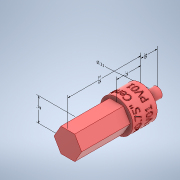
# Autodesk Inventor part: 1x8mmx1_75-inchHexShaft
Saved by Autodesk Inventor 2022.2 (Build 262287000, 287)
## iProperties
Created: 2020-11-16
Part Number: 1x8mmx1_75-inchHexShaft
Material: PC/ABS Plastic
Document SubType Name: Modeling
Designer: robst
Density: 0.357273 g/cm^3
Appearance: Smooth - Red
Author: robst
Autodesk Inventor part; units mm, degrees
ref_plane "XZ Plane" through (0, 0, 0) normal (0, 1, 0) x (-1, 0, 0)
ref_plane "XY Plane" through (0, 0, 0) normal (0, 0, 1) x (1, 0, 0)
sketch "Sketch1" plane through (0, 0, 0) normal (0, 0, 1) x (1, 0, 0)
  line L0 (10.9985, 0) -> (5.4993, -9.525)
  line L1 (5.4993, -9.525) -> (-5.4993, -9.525)
  line L2 (-5.4993, -9.525) -> (-10.9985, 0)
  line L3 (-10.9985, 0) -> (-5.4993, 9.525)
  line L4 (-5.4993, 9.525) -> (5.4993, 9.525)
  line L5 (5.4993, 9.525) -> (10.9985, 0)
  point P0 (0, 0)
  point P1 (0, 0)
  dimension "d0" = 19.05
  constraints: 12 end point, 1 coincident, 1 horizontal, 13 other
  measures "d0" distance between parallel lines of L1 L4
extrude "Hex Portion" add sketch "Sketch1" along normal mid plane 38.1
sketch "Sketch2" plane through (0, 0, -19.05) normal (0, 0, -1) x (-1, 0, 0)
  circle A0 centre (0, 0) radius 12.7
  dimension "d3" = 25.4
  constraints: 1 centre point, 1 coincident
  measures "d3" diameter of A0
extrude "Extrusion2" add sketch "Sketch2" along normal blind 19.05
thicken "Reduce Size of Hex Shaft" operation add thickness 0.1905 both sides no extend neighbours yes toward (-0.8660254, -0.5, 0) faces at (9.1654, 3.175, -6.35) (-1.8331, 9.525, 6.35) (7.3323, -6.35, -6.35) (-1.8331, -9.525, -6.35) (-7.3323, -6.35, 6.35) (-9.1654, 3.175, 6.35)
sketch "Sketch3" plane through (0, 0, -38.1) normal (0, 0, -1) x (-1, 0, 0)
  circle A0 centre (0, 0) radius 4
  dimension "d14" = 8
  constraints: 1 centre point, 1 coincident
  measures "d14" diameter of A0
extrude "Extrusion3" add sketch "Sketch3" along normal blind 12.7
ref_plane "Work Plane1" through (12.7, 0, -19.05) normal (1, 0, 0) x (0, 1, 0)
sketch "Sketch4" plane through (12.7, 0, -19.05) normal (1, 0, 0) x (0, 1, 0)
  line L0 (-12.7, 0) -> (12.7, 0) projected
  line L1 (-12.7, -19.05) -> (12.7, -19.05) projected
  line L2 (-12.7, 0) -> (-12.7, -19.05) construction
  line L3 (-12.7, -9.525) -> (12.7, -9.525) construction
  line L4 (12.7, 0) -> (12.7, -19.05) construction
  line L5 (-30.7085, -6.985) -> (-33.1867, -6.985)
  line L6 (-33.1867, -6.985) -> (-33.1867, -6.4663)
  line L7 (-33.1867, -6.4663) -> (-32.2646, -6.4663)
  line L8 (-32.2646, -6.4663) -> (-32.2646, -3.0618)
  line L9 (-32.2646, -3.0618) -> (-33.1867, -3.0618)
  line L10 (-33.1867, -3.0618) -> (-33.1867, -2.5966)
  spline S0 degree 2 poles (-33.1867, -2.5966) (-32.6639, -2.5966) (-32.1699, -2.3002) (-32.137, -1.8885) knots 0 0 0 1 2 2 2
  line L11 (-32.137, -1.8885) -> (-31.61, -1.8885)
  line L12 (-31.61, -1.8885) -> (-31.61, -6.4663)
  line L13 (-31.61, -6.4663) -> (-30.7085, -6.4663)
  line L14 (-30.7085, -6.4663) -> (-30.7085, -6.985)
  line L15 (-29.0124, -1.6786) -> (-29.1606, -3.6546)
  line L16 (-29.1606, -3.6546) -> (-29.6093, -3.6546)
  line L17 (-29.6093, -3.6546) -> (-29.7575, -1.6786)
  line L18 (-29.7575, -1.6786) -> (-29.0124, -1.6786)
  line L19 (-27.728, -1.6786) -> (-27.8762, -3.6546)
  line L20 (-27.8762, -3.6546) -> (-28.3249, -3.6546)
  line L21 (-28.3249, -3.6546) -> (-28.4731, -1.6786)
  line L22 (-28.4731, -1.6786) -> (-27.728, -1.6786)
  line L23 (-23.9159, -6.985) -> (-24.7022, -6.985)
  line L24 (-24.7022, -6.985) -> (-25.6285, -5.5524)
  line L25 (-25.6285, -5.5524) -> (-26.5794, -6.985)
  line L26 (-26.5794, -6.985) -> (-27.3081, -6.985)
  line L27 (-27.3081, -6.985) -> (-25.9866, -5.0954)
  line L28 (-25.9866, -5.0954) -> (-27.2957, -3.1729)
  line L29 (-27.2957, -3.1729) -> (-26.5095, -3.1729)
  line L30 (-26.5095, -3.1729) -> (-25.5873, -4.5932)
  line L31 (-25.5873, -4.5932) -> (-24.6446, -3.1729)
  line L32 (-24.6446, -3.1729) -> (-23.9159, -3.1729)
  line L33 (-23.9159, -3.1729) -> (-25.2292, -5.0543)
  line L34 (-25.2292, -5.0543) -> (-23.9159, -6.985)
  spline S1 degree 2 poles (-21.977, -7.1003) (-22.3557, -7.1003) (-22.9773, -6.8738) (-23.1955, -6.6639) knots 0 0 0 1 2 2 2
  spline S2 degree 2 poles (-23.1955, -6.6639) (-23.4096, -6.4581) (-23.6319, -5.8982) (-23.6319, -5.5812) knots 0 0 0 1 2 2 2
  spline S3 degree 2 poles (-23.6319, -5.5812) (-23.6319, -5.1695) (-23.1914, -4.4779) (-22.7715, -4.2721) knots 0 0 0 1 2 2 2
  line L35 (-22.7715, -4.2721) -> (-22.7715, -4.2515)
  spline S4 degree 2 poles (-22.7715, -4.2515) (-23.1461, -4.0333) (-23.5084, -3.5146) (-23.5084, -3.1277) knots 0 0 0 1 2 2 2
  spline S5 degree 2 poles (-23.5084, -3.1277) (-23.5084, -2.5554) (-22.6439, -1.7897) (-21.977, -1.7897) knots 0 0 0 1 2 2 2
  spline S6 degree 2 poles (-21.977, -1.7897) (-21.2854, -1.7897) (-20.4497, -2.5143) (-20.4497, -3.0824) knots 0 0 0 1 2 2 2
  spline S7 degree 2 poles (-20.4497, -3.0824) (-20.4497, -3.4241) (-20.849, -4.091) (-21.2236, -4.2803) knots 0 0 0 1 2 2 2
  line L36 (-21.2236, -4.2803) -> (-21.2236, -4.3009)
  spline S8 degree 2 poles (-21.2236, -4.3009) (-20.779, -4.5068) (-20.3221, -5.0996) (-20.3221, -5.5689) knots 0 0 0 1 2 2 2
  spline S9 degree 2 poles (-20.3221, -5.5689) (-20.3221, -6.2193) (-21.2689, -7.1003) (-21.977, -7.1003) knots 0 0 0 1 2 2 2
  spline S10 degree 2 poles (-21.0219, -5.6347) (-21.0219, -5.3219) (-21.2689, -4.9514) (-21.6188, -4.762) knots 0 0 0 1 2 2 2
  spline S11 degree 2 poles (-21.6188, -4.762) (-21.7341, -4.6961) (-22.1211, -4.5438) (-22.3639, -4.445) knots 0 0 0 1 2 2 2
  spline S12 degree 2 poles (-22.3639, -4.445) (-22.6439, -4.6303) (-22.9444, -5.1819) (-22.9444, -5.5318) knots 0 0 0 1 2 2 2
  spline S13 degree 2 poles (-22.9444, -5.5318) (-22.9444, -5.9929) (-22.3886, -6.5939) (-21.9687, -6.5939) knots 0 0 0 1 2 2 2
  spline S14 degree 2 poles (-21.9687, -6.5939) (-21.5406, -6.5939) (-21.0219, -6.0793) (-21.0219, -5.6347) knots 0 0 0 1 2 2 2
  spline S15 degree 2 poles (-21.1166, -3.0906) (-21.1166, -2.7489) (-21.5735, -2.292) (-21.9811, -2.292) knots 0 0 0 1 2 2 2
  spline S16 degree 2 poles (-21.9811, -2.292) (-22.3516, -2.292) (-22.825, -2.6995) (-22.825, -3.0494) knots 0 0 0 1 2 2 2
  spline S17 degree 2 poles (-22.825, -3.0494) (-22.825, -3.3006) (-22.5821, -3.6505) (-22.3392, -3.7904) knots 0 0 0 1 2 2 2
  spline S18 degree 2 poles (-22.3392, -3.7904) (-22.2363, -3.8481) (-21.8, -4.0498) (-21.6229, -4.1074) knots 0 0 0 1 2 2 2
  spline S19 degree 2 poles (-21.6229, -4.1074) (-21.3265, -3.881) (-21.1166, -3.3994) (-21.1166, -3.0906) knots 0 0 0 1 2 2 2
  line L37 (-15.2832, -6.985) -> (-15.2832, -4.7785)
  spline S20 degree 2 poles (-15.2832, -4.7785) (-15.2832, -4.515) (-15.3244, -4.0663) (-15.3903, -3.9428) knots 0 0 0 1 2 2 2
  spline S21 degree 2 poles (-15.3903, -3.9428) (-15.4561, -3.8069) (-15.7072, -3.6752) (-15.9254, -3.6752) knots 0 0 0 1 2 2 2
  spline S22 degree 2 poles (-15.9254, -3.6752) (-16.123, -3.6752) (-16.5759, -3.9181) (-16.8146, -4.1486) knots 0 0 0 1 2 2 2
  spline S23 degree 2 poles (-16.8146, -4.1486) (-16.8105, -4.2062) (-16.8023, -4.3668) (-16.8023, -4.4738) knots 0 0 0 1 2 2 2
  line L38 (-16.8023, -4.4738) -> (-16.8023, -6.985)
  line L39 (-16.8023, -6.985) -> (-17.4445, -6.985)
  line L40 (-17.4445, -6.985) -> (-17.4445, -4.7785)
  spline S24 degree 2 poles (-17.4445, -4.7785) (-17.4445, -4.515) (-17.4857, -4.0663) (-17.5515, -3.9428) knots 0 0 0 1 2 2 2
  spline S25 degree 2 poles (-17.5515, -3.9428) (-17.6174, -3.8069) (-17.8685, -3.6752) (-18.0867, -3.6752) knots 0 0 0 1 2 2 2
  spline S26 degree 2 poles (-18.0867, -3.6752) (-18.2925, -3.6752) (-18.7495, -3.9345) (-18.9636, -4.1362) knots 0 0 0 1 2 2 2
  line L41 (-18.9636, -4.1362) -> (-18.9636, -6.985)
  line L42 (-18.9636, -6.985) -> (-19.6058, -6.985)
  line L43 (-19.6058, -6.985) -> (-19.6058, -3.1729)
  line L44 (-19.6058, -3.1729) -> (-18.9636, -3.1729)
  line L45 (-18.9636, -3.1729) -> (-18.9636, -3.5928)
  spline S27 degree 2 poles (-18.9636, -3.5928) (-18.7124, -3.3417) (-18.2184, -3.0659) (-17.922, -3.0659) knots 0 0 0 1 2 2 2
  spline S28 degree 2 poles (-17.922, -3.0659) (-17.5845, -3.0659) (-17.0616, -3.3747) (-16.9258, -3.7246) knots 0 0 0 1 2 2 2
  spline S29 degree 2 poles (-16.9258, -3.7246) (-16.6335, -3.3994) (-16.0819, -3.0659) (-15.7608, -3.0659) knots 0 0 0 1 2 2 2
  spline S30 degree 2 poles (-15.7608, -3.0659) (-15.5138, -3.0659) (-15.1103, -3.2182) (-14.9621, -3.3911) knots 0 0 0 1 2 2 2
  spline S31 degree 2 poles (-14.9621, -3.3911) (-14.8098, -3.564) (-14.641, -4.0827) (-14.641, -4.4738) knots 0 0 0 1 2 2 2
  line L46 (-14.641, -4.4738) -> (-14.641, -6.985)
  line L47 (-14.641, -6.985) -> (-15.2832, -6.985)
  line L48 (-9.4169, -6.985) -> (-9.4169, -4.7785)
  spline S32 degree 2 poles (-9.4169, -4.7785) (-9.4169, -4.515) (-9.4581, -4.0663) (-9.524, -3.9428) knots 0 0 0 1 2 2 2
  spline S33 degree 2 poles (-9.524, -3.9428) (-9.5898, -3.8069) (-9.841, -3.6752) (-10.0591, -3.6752) knots 0 0 0 1 2 2 2
  spline S34 degree 2 poles (-10.0591, -3.6752) (-10.2567, -3.6752) (-10.7096, -3.9181) (-10.9483, -4.1486) knots 0 0 0 1 2 2 2
  spline S35 degree 2 poles (-10.9483, -4.1486) (-10.9442, -4.2062) (-10.936, -4.3668) (-10.936, -4.4738) knots 0 0 0 1 2 2 2
  line L49 (-10.936, -4.4738) -> (-10.936, -6.985)
  line L50 (-10.936, -6.985) -> (-11.5782, -6.985)
  line L51 (-11.5782, -6.985) -> (-11.5782, -4.7785)
  spline S36 degree 2 poles (-11.5782, -4.7785) (-11.5782, -4.515) (-11.6194, -4.0663) (-11.6852, -3.9428) knots 0 0 0 1 2 2 2
  spline S37 degree 2 poles (-11.6852, -3.9428) (-11.7511, -3.8069) (-12.0022, -3.6752) (-12.2204, -3.6752) knots 0 0 0 1 2 2 2
  spline S38 degree 2 poles (-12.2204, -3.6752) (-12.4262, -3.6752) (-12.8832, -3.9345) (-13.0973, -4.1362) knots 0 0 0 1 2 2 2
  line L52 (-13.0973, -4.1362) -> (-13.0973, -6.985)
  line L53 (-13.0973, -6.985) -> (-13.7395, -6.985)
  line L54 (-13.7395, -6.985) -> (-13.7395, -3.1729)
  line L55 (-13.7395, -3.1729) -> (-13.0973, -3.1729)
  line L56 (-13.0973, -3.1729) -> (-13.0973, -3.5928)
  spline S39 degree 2 poles (-13.0973, -3.5928) (-12.8461, -3.3417) (-12.3521, -3.0659) (-12.0557, -3.0659) knots 0 0 0 1 2 2 2
  spline S40 degree 2 poles (-12.0557, -3.0659) (-11.7182, -3.0659) (-11.1953, -3.3747) (-11.0595, -3.7246) knots 0 0 0 1 2 2 2
  spline S41 degree 2 poles (-11.0595, -3.7246) (-10.7672, -3.3994) (-10.2156, -3.0659) (-9.8945, -3.0659) knots 0 0 0 1 2 2 2
  spline S42 degree 2 poles (-9.8945, -3.0659) (-9.6475, -3.0659) (-9.244, -3.2182) (-9.0958, -3.3911) knots 0 0 0 1 2 2 2
  spline S43 degree 2 poles (-9.0958, -3.3911) (-8.9435, -3.564) (-8.7747, -4.0827) (-8.7747, -4.4738) knots 0 0 0 1 2 2 2
  line L57 (-8.7747, -4.4738) -> (-8.7747, -6.985)
  line L58 (-8.7747, -6.985) -> (-9.4169, -6.985)
  line L59 (-4.9133, -6.985) -> (-5.6996, -6.985)
  line L60 (-5.6996, -6.985) -> (-6.6258, -5.5524)
  line L61 (-6.6258, -5.5524) -> (-7.5768, -6.985)
  line L62 (-7.5768, -6.985) -> (-8.3054, -6.985)
  line L63 (-8.3054, -6.985) -> (-6.984, -5.0954)
  line L64 (-6.984, -5.0954) -> (-8.2931, -3.1729)
  line L65 (-8.2931, -3.1729) -> (-7.5068, -3.1729)
  line L66 (-7.5068, -3.1729) -> (-6.5847, -4.5932)
  line L67 (-6.5847, -4.5932) -> (-5.6419, -3.1729)
  line L68 (-5.6419, -3.1729) -> (-4.9133, -3.1729)
  line L69 (-4.9133, -3.1729) -> (-6.2265, -5.0543)
  line L70 (-6.2265, -5.0543) -> (-4.9133, -6.985)
  spline S44 degree 2 poles (-1.3482, -4.445) (-1.3482, -5.8117) (-2.1427, -7.092) (-2.9702, -7.092) knots 0 0 0 1 2 2 2
  spline S45 degree 2 poles (-2.9702, -7.092) (-3.81, -7.092) (-4.5963, -5.787) (-4.5963, -4.4491) knots 0 0 0 1 2 2 2
  spline S46 degree 2 poles (-4.5963, -4.4491) (-4.5963, -3.0741) (-3.8018, -1.8021) (-2.9702, -1.8021) knots 0 0 0 1 2 2 2
  spline S47 degree 2 poles (-2.9702, -1.8021) (-2.1345, -1.8021) (-1.3482, -3.1194) (-1.3482, -4.445) knots 0 0 0 1 2 2 2
  spline S48 degree 2 poles (-2.221, -5.9929) (-2.1222, -5.7418) (-2.0398, -4.9678) (-2.0398, -4.445) knots 0 0 0 1 2 2 2
  spline S49 degree 2 poles (-2.0398, -4.445) (-2.0398, -3.9222) (-2.1222, -3.1524) (-2.2251, -2.893) knots 0 0 0 1 2 2 2
  spline S50 degree 2 poles (-2.2251, -2.893) (-2.328, -2.6337) (-2.6861, -2.3661) (-2.9702, -2.3661) knots 0 0 0 1 2 2 2
  spline S51 degree 2 poles (-2.9702, -2.3661) (-3.2542, -2.3661) (-3.6206, -2.6337) (-3.7277, -2.9012) knots 0 0 0 1 2 2 2
  spline S52 degree 2 poles (-3.7277, -2.9012) (-3.8306, -3.1606) (-3.9047, -3.951) (-3.9047, -4.4491) knots 0 0 0 1 2 2 2
  spline S53 degree 2 poles (-3.9047, -4.4491) (-3.9047, -4.9843) (-3.8388, -5.7006) (-3.7318, -5.9805) knots 0 0 0 1 2 2 2
  spline S54 degree 2 poles (-3.7318, -5.9805) (-3.633, -6.244) (-3.2666, -6.528) (-2.9702, -6.528) knots 0 0 0 1 2 2 2
  spline S55 degree 2 poles (-2.9702, -6.528) (-2.6903, -6.528) (-2.3239, -6.2605) (-2.221, -5.9929) knots 0 0 0 1 2 2 2
  line L71 (0.3931, -6.985) -> (-0.422, -6.985)
  line L72 (-0.422, -6.985) -> (-0.422, -6.0135)
  line L73 (-0.422, -6.0135) -> (0.3931, -6.0135)
  line L74 (0.3931, -6.0135) -> (0.3931, -6.985)
  line L75 (4.6086, -2.6666) -> (2.4103, -6.985)
  line L76 (2.4103, -6.985) -> (1.6858, -6.985)
  line L77 (1.6858, -6.985) -> (4.0076, -2.5019)
  line L78 (4.0076, -2.5019) -> (1.3853, -2.5019)
  line L79 (1.3853, -2.5019) -> (1.3853, -1.905)
  line L80 (1.3853, -1.905) -> (4.6086, -1.905)
  line L81 (4.6086, -1.905) -> (4.6086, -2.6666)
  spline S56 degree 2 poles (8.3095, -5.3713) (8.3095, -5.7376) (8.0749, -6.3634) (7.8608, -6.5939) knots 0 0 0 1 2 2 2
  spline S57 degree 2 poles (7.8608, -6.5939) (7.6468, -6.8244) (7.0087, -7.092) (6.6135, -7.092) knots 0 0 0 1 2 2 2
  spline S58 degree 2 poles (6.6135, -7.092) (6.2512, -7.092) (5.5431, -6.9315) (5.2838, -6.8039) knots 0 0 0 1 2 2 2
  line L82 (5.2838, -6.8039) -> (5.2838, -6.0834)
  line L83 (5.2838, -6.0834) -> (5.3332, -6.0834)
  spline S59 degree 2 poles (5.3332, -6.0834) (5.4114, -6.1411) (5.7037, -6.2893) (5.8807, -6.3551) knots 0 0 0 1 2 2 2
  spline S60 degree 2 poles (5.8807, -6.3551) (6.0824, -6.4251) (6.4159, -6.5033) (6.6258, -6.5033) knots 0 0 0 1 2 2 2
  spline S61 degree 2 poles (6.6258, -6.5033) (6.8317, -6.5033) (7.2186, -6.3551) (7.3586, -6.1946) knots 0 0 0 1 2 2 2
  spline S62 degree 2 poles (7.3586, -6.1946) (7.4862, -6.0423) (7.6179, -5.6388) (7.6179, -5.3671) knots 0 0 0 1 2 2 2
  spline S63 degree 2 poles (7.6179, -5.3671) (7.6179, -5.0954) (7.4697, -4.7496) (7.3298, -4.6344) knots 0 0 0 1 2 2 2
  spline S64 degree 2 poles (7.3298, -4.6344) (7.1857, -4.5068) (6.7576, -4.3997) (6.4982, -4.3997) knots 0 0 0 1 2 2 2
  spline S65 degree 2 poles (6.4982, -4.3997) (6.2183, -4.3997) (5.6625, -4.4862) (5.4937, -4.5232) knots 0 0 0 1 2 2 2
  line L84 (5.4937, -4.5232) -> (5.4937, -1.905)
  line L85 (5.4937, -1.905) -> (8.2807, -1.905)
  line L86 (8.2807, -1.905) -> (8.2807, -2.5019)
  line L87 (8.2807, -2.5019) -> (6.1483, -2.5019)
  line L88 (6.1483, -2.5019) -> (6.1483, -3.8563)
  spline S66 degree 2 poles (6.1483, -3.8563) (6.2718, -3.8398) (6.5105, -3.8275) (6.6094, -3.8275) knots 0 0 0 1 2 2 2
  spline S67 degree 2 poles (6.6094, -3.8275) (7.0004, -3.8275) (7.5397, -3.9551) (7.7867, -4.1445) knots 0 0 0 1 2 2 2
  spline S68 degree 2 poles (7.7867, -4.1445) (8.0378, -4.3338) (8.3095, -4.9102) (8.3095, -5.3713) knots 0 0 0 1 2 2 2
  line L89 (9.8039, -1.6786) -> (9.6557, -3.6546)
  line L90 (9.6557, -3.6546) -> (9.207, -3.6546)
  line L91 (9.207, -3.6546) -> (9.0588, -1.6786)
  line L92 (9.0588, -1.6786) -> (9.8039, -1.6786)
  line L93 (11.0883, -1.6786) -> (10.9401, -3.6546)
  line L94 (10.9401, -3.6546) -> (10.4914, -3.6546)
  line L95 (10.4914, -3.6546) -> (10.3432, -1.6786)
  line L96 (10.3432, -1.6786) -> (11.0883, -1.6786)
  spline S69 degree 2 poles (16.156, -7.0756) (15.662, -7.0756) (14.8263, -6.7421) (14.5216, -6.4087) knots 0 0 0 1 2 2 2
  spline S70 degree 2 poles (14.5216, -6.4087) (14.217, -6.0793) (13.8835, -5.0913) (13.8835, -4.4491) knots 0 0 0 1 2 2 2
  spline S71 degree 2 poles (13.8835, -4.4491) (13.8835, -3.811) (14.2088, -2.8642) (14.5175, -2.5143) knots 0 0 0 1 2 2 2
  spline S72 degree 2 poles (14.5175, -2.5143) (14.8222, -2.1726) (15.6537, -1.8144) (16.1683, -1.8144) knots 0 0 0 1 2 2 2
  spline S73 degree 2 poles (16.1683, -1.8144) (16.4235, -1.8144) (16.8723, -1.8885) (17.0616, -1.9462) knots 0 0 0 1 2 2 2
  spline S74 degree 2 poles (17.0616, -1.9462) (17.2263, -1.9997) (17.568, -2.152) (17.7368, -2.2426) knots 0 0 0 1 2 2 2
  line L97 (17.7368, -2.2426) -> (17.7368, -3.0577)
  line L98 (17.7368, -3.0577) -> (17.6833, -3.0577)
  spline S75 degree 2 poles (17.6833, -3.0577) (17.5927, -2.9753) (17.3128, -2.7448) (17.111, -2.6337) knots 0 0 0 1 2 2 2
  spline S76 degree 2 poles (17.111, -2.6337) (16.9176, -2.5266) (16.4606, -2.3908) (16.1642, -2.3908) knots 0 0 0 1 2 2 2
  spline S77 degree 2 poles (16.1642, -2.3908) (15.839, -2.3908) (15.2585, -2.6584) (15.0403, -2.9136) knots 0 0 0 1 2 2 2
  spline S78 degree 2 poles (15.0403, -2.9136) (14.8263, -3.1729) (14.5875, -3.9592) (14.5875, -4.4491) knots 0 0 0 1 2 2 2
  spline S79 degree 2 poles (14.5875, -4.4491) (14.5875, -4.9719) (14.8386, -5.7253) (15.0568, -5.9846) knots 0 0 0 1 2 2 2
  spline S80 degree 2 poles (15.0568, -5.9846) (15.2709, -6.2358) (15.8431, -6.491) (16.1642, -6.491) knots 0 0 0 1 2 2 2
  spline S81 degree 2 poles (16.1642, -6.491) (16.4565, -6.491) (16.9546, -6.3469) (17.1481, -6.2399) knots 0 0 0 1 2 2 2
  spline S82 degree 2 poles (17.1481, -6.2399) (17.3333, -6.1328) (17.6092, -5.9105) (17.6874, -5.8323) knots 0 0 0 1 2 2 2
  line L99 (17.6874, -5.8323) -> (17.7368, -5.8323)
  line L100 (17.7368, -5.8323) -> (17.7368, -6.6392)
  spline S83 degree 2 poles (17.7368, -6.6392) (17.568, -6.7174) (17.2716, -6.8615) (17.0616, -6.9274) knots 0 0 0 1 2 2 2
  spline S84 degree 2 poles (17.0616, -6.9274) (16.8393, -7.0015) (16.4606, -7.0756) (16.156, -7.0756) knots 0 0 0 1 2 2 2
  spline S85 degree 2 poles (19.9721, -7.0715) (19.0582, -7.0715) (18.0538, -6.0464) (18.0538, -5.0996) knots 0 0 0 1 2 2 2
  spline S86 degree 2 poles (18.0538, -5.0996) (18.0538, -4.1692) (19.0294, -3.0659) (19.8157, -3.0659) knots 0 0 0 1 2 2 2
  spline S87 degree 2 poles (19.8157, -3.0659) (20.1697, -3.0659) (20.7173, -3.2717) (20.919, -3.4899) knots 0 0 0 1 2 2 2
  spline S88 degree 2 poles (20.919, -3.4899) (21.1248, -3.7081) (21.343, -4.338) (21.343, -4.7949) knots 0 0 0 1 2 2 2
  line L101 (21.343, -4.7949) -> (21.343, -5.1448)
  line L102 (21.343, -5.1448) -> (18.7042, -5.1448)
  spline S89 degree 2 poles (18.7042, -5.1448) (18.7042, -5.8076) (19.3711, -6.5116) (19.9639, -6.5116) knots 0 0 0 1 2 2 2
  spline S90 degree 2 poles (19.9639, -6.5116) (20.1739, -6.5116) (20.5814, -6.4169) (20.7461, -6.3428) knots 0 0 0 1 2 2 2
  spline S91 degree 2 poles (20.7461, -6.3428) (20.919, -6.2605) (21.1577, -6.1164) (21.236, -6.0505) knots 0 0 0 1 2 2 2
  line L103 (21.236, -6.0505) -> (21.273, -6.0505)
  line L104 (21.273, -6.0505) -> (21.273, -6.7503)
  spline S92 degree 2 poles (21.273, -6.7503) (21.1619, -6.7956) (20.8243, -6.9274) (20.6926, -6.9644) knots 0 0 0 1 2 2 2
  spline S93 degree 2 poles (20.6926, -6.9644) (20.5073, -7.0179) (20.2027, -7.0715) (19.9721, -7.0715) knots 0 0 0 1 2 2 2
  spline S94 degree 2 poles (20.7173, -4.655) (20.709, -4.3956) (20.602, -4.0169) (20.4991, -3.8892) knots 0 0 0 1 2 2 2
  spline S95 degree 2 poles (20.4991, -3.8892) (20.3879, -3.7452) (20.038, -3.5928) (19.7787, -3.5928) knots 0 0 0 1 2 2 2
  spline S96 degree 2 poles (19.7787, -3.5928) (19.5234, -3.5928) (19.1653, -3.7452) (19.0171, -3.8934) knots 0 0 0 1 2 2 2
  spline S97 degree 2 poles (19.0171, -3.8934) (18.873, -4.0457) (18.7248, -4.4121) (18.7042, -4.655) knots 0 0 0 1 2 2 2
  line L105 (18.7042, -4.655) -> (20.7173, -4.655)
  line L106 (24.9863, -6.985) -> (24.3441, -6.985)
  line L107 (24.3441, -6.985) -> (24.3441, -4.8114)
  spline S98 degree 2 poles (24.3441, -4.8114) (24.3441, -4.5479) (24.2947, -4.0951) (24.2206, -3.9592) knots 0 0 0 1 2 2 2
  spline S99 degree 2 poles (24.2206, -3.9592) (24.1423, -3.8151) (23.8624, -3.6752) (23.6236, -3.6752) knots 0 0 0 1 2 2 2
  spline S100 degree 2 poles (23.6236, -3.6752) (23.3849, -3.6752) (22.8785, -3.9304) (22.6356, -4.1362) knots 0 0 0 1 2 2 2
  line L108 (22.6356, -4.1362) -> (22.6356, -6.985)
  line L109 (22.6356, -6.985) -> (21.9934, -6.985)
  line L110 (21.9934, -6.985) -> (21.9934, -3.1729)
  line L111 (21.9934, -3.1729) -> (22.6356, -3.1729)
  line L112 (22.6356, -3.1729) -> (22.6356, -3.597)
  spline S101 degree 2 poles (22.6356, -3.597) (22.9238, -3.3376) (23.4796, -3.0659) (23.7924, -3.0659) knots 0 0 0 1 2 2 2
  spline S102 degree 2 poles (23.7924, -3.0659) (24.3523, -3.0659) (24.9863, -3.8069) (24.9863, -4.5109) knots 0 0 0 1 2 2 2
  line L113 (24.9863, -4.5109) -> (24.9863, -6.985)
  spline S103 degree 2 poles (27.0405, -7.0591) (26.5177, -7.0591) (25.929, -6.4622) (25.929, -5.8159) knots 0 0 0 1 2 2 2
  line L114 (25.929, -5.8159) -> (25.929, -3.704)
  line L115 (25.929, -3.704) -> (25.4967, -3.704)
  line L116 (25.4967, -3.704) -> (25.4967, -3.1729)
  line L117 (25.4967, -3.1729) -> (25.929, -3.1729)
  line L118 (25.929, -3.1729) -> (25.929, -2.0779)
  line L119 (25.929, -2.0779) -> (26.5712, -2.0779)
  line L120 (26.5712, -2.0779) -> (26.5712, -3.1729)
  line L121 (26.5712, -3.1729) -> (27.7527, -3.1729)
  line L122 (27.7527, -3.1729) -> (27.7527, -3.704)
  line L123 (27.7527, -3.704) -> (26.5712, -3.704)
  line L124 (26.5712, -3.704) -> (26.5712, -5.5195)
  spline S104 degree 2 poles (26.5712, -5.5195) (26.5712, -5.8076) (26.5918, -6.1246) (26.6618, -6.2605) knots 0 0 0 1 2 2 2
  spline S105 degree 2 poles (26.6618, -6.2605) (26.7194, -6.3798) (26.9788, -6.4992) (27.2011, -6.4992) knots 0 0 0 1 2 2 2
  spline S106 degree 2 poles (27.2011, -6.4992) (27.3575, -6.4992) (27.6498, -6.4045) (27.7156, -6.3757) knots 0 0 0 1 2 2 2
  line L125 (27.7156, -6.3757) -> (27.7527, -6.3757)
  line L126 (27.7527, -6.3757) -> (27.7527, -6.9521)
  spline S107 degree 2 poles (27.7527, -6.9521) (27.5716, -7.0015) (27.2011, -7.0591) (27.0405, -7.0591) knots 0 0 0 1 2 2 2
  spline S108 degree 2 poles (29.881, -7.0715) (28.9671, -7.0715) (27.9626, -6.0464) (27.9626, -5.0996) knots 0 0 0 1 2 2 2
  spline S109 degree 2 poles (27.9626, -5.0996) (27.9626, -4.1692) (28.9383, -3.0659) (29.7246, -3.0659) knots 0 0 0 1 2 2 2
  spline S110 degree 2 poles (29.7246, -3.0659) (30.0786, -3.0659) (30.6261, -3.2717) (30.8279, -3.4899) knots 0 0 0 1 2 2 2
  spline S111 degree 2 poles (30.8279, -3.4899) (31.0337, -3.7081) (31.2519, -4.338) (31.2519, -4.7949) knots 0 0 0 1 2 2 2
  line L127 (31.2519, -4.7949) -> (31.2519, -5.1448)
  line L128 (31.2519, -5.1448) -> (28.6131, -5.1448)
  spline S112 degree 2 poles (28.6131, -5.1448) (28.6131, -5.8076) (29.28, -6.5116) (29.8728, -6.5116) knots 0 0 0 1 2 2 2
  spline S113 degree 2 poles (29.8728, -6.5116) (30.0827, -6.5116) (30.4903, -6.4169) (30.655, -6.3428) knots 0 0 0 1 2 2 2
  spline S114 degree 2 poles (30.655, -6.3428) (30.8279, -6.2605) (31.0666, -6.1164) (31.1448, -6.0505) knots 0 0 0 1 2 2 2
  line L129 (31.1448, -6.0505) -> (31.1819, -6.0505)
  line L130 (31.1819, -6.0505) -> (31.1819, -6.7503)
  spline S115 degree 2 poles (31.1819, -6.7503) (31.0707, -6.7956) (30.7332, -6.9274) (30.6014, -6.9644) knots 0 0 0 1 2 2 2
  spline S116 degree 2 poles (30.6014, -6.9644) (30.4162, -7.0179) (30.1116, -7.0715) (29.881, -7.0715) knots 0 0 0 1 2 2 2
  spline S117 degree 2 poles (30.6261, -4.655) (30.6179, -4.3956) (30.5109, -4.0169) (30.408, -3.8892) knots 0 0 0 1 2 2 2
  spline S118 degree 2 poles (30.408, -3.8892) (30.2968, -3.7452) (29.9469, -3.5928) (29.6875, -3.5928) knots 0 0 0 1 2 2 2
  spline S119 degree 2 poles (29.6875, -3.5928) (29.4323, -3.5928) (29.0741, -3.7452) (28.9259, -3.8934) knots 0 0 0 1 2 2 2
  spline S120 degree 2 poles (28.9259, -3.8934) (28.7819, -4.0457) (28.6337, -4.4121) (28.6131, -4.655) knots 0 0 0 1 2 2 2
  line L131 (28.6131, -4.655) -> (30.6261, -4.655)
  line L132 (33.9236, -3.8604) -> (33.8907, -3.8604)
  spline S121 degree 2 poles (33.8907, -3.8604) (33.8166, -3.8398) (33.656, -3.8316) (33.5449, -3.8316) knots 0 0 0 1 2 2 2
  spline S122 degree 2 poles (33.5449, -3.8316) (33.2855, -3.8316) (32.7751, -4.058) (32.5445, -4.2803) knots 0 0 0 1 2 2 2
  line L133 (32.5445, -4.2803) -> (32.5445, -6.985)
  line L134 (32.5445, -6.985) -> (31.9023, -6.985)
  line L135 (31.9023, -6.985) -> (31.9023, -3.1729)
  line L136 (31.9023, -3.1729) -> (32.5445, -3.1729)
  line L137 (32.5445, -3.1729) -> (32.5445, -3.741)
  spline S123 degree 2 poles (32.5445, -3.741) (32.8944, -3.4282) (33.4173, -3.1729) (33.6643, -3.1729) knots 0 0 0 1 2 2 2
  spline S124 degree 2 poles (33.6643, -3.1729) (33.7631, -3.1729) (33.8619, -3.1812) (33.9236, -3.1935) knots 0 0 0 1 2 2 2
  line L138 (33.9236, -3.1935) -> (33.9236, -3.8604)
  spline S125 degree 2 poles (-21.979, -15.6168) (-22.5307, -15.6168) (-23.3046, -15.3863) (-23.6463, -15.2216) knots 0 0 0 1 2 2 2
  line L139 (-23.6463, -15.2216) -> (-23.6463, -14.3735)
  line L140 (-23.6463, -14.3735) -> (-23.5969, -14.3735)
  spline S126 degree 2 poles (-23.5969, -14.3735) (-23.2634, -14.6864) (-22.4195, -15.0322) (-22.0284, -15.0322) knots 0 0 0 1 2 2 2
  spline S127 degree 2 poles (-22.0284, -15.0322) (-21.4686, -15.0322) (-20.8963, -14.567) (-20.8963, -14.1842) knots 0 0 0 1 2 2 2
  spline S128 degree 2 poles (-20.8963, -14.1842) (-20.8963, -13.8795) (-21.1969, -13.5008) (-21.5221, -13.4061) knots 0 0 0 1 2 2 2
  spline S129 degree 2 poles (-21.5221, -13.4061) (-21.7567, -13.3403) (-22.1478, -13.2497) (-22.4401, -13.1756) knots 0 0 0 1 2 2 2
  spline S130 degree 2 poles (-22.4401, -13.1756) (-22.7036, -13.1056) (-23.1194, -12.8957) (-23.2799, -12.7269) knots 0 0 0 1 2 2 2
  spline S131 degree 2 poles (-23.2799, -12.7269) (-23.4363, -12.5581) (-23.6092, -12.1053) (-23.6092, -11.8088) knots 0 0 0 1 2 2 2
  spline S132 degree 2 poles (-23.6092, -11.8088) (-23.6092, -11.1913) (-22.6459, -10.3557) (-21.9008, -10.3557) knots 0 0 0 1 2 2 2
  spline S133 degree 2 poles (-21.9008, -10.3557) (-21.4727, -10.3557) (-20.7152, -10.5244) (-20.39, -10.685) knots 0 0 0 1 2 2 2
  line L141 (-20.39, -10.685) -> (-20.39, -11.4919)
  line L142 (-20.39, -11.4919) -> (-20.4394, -11.4919)
  spline S134 degree 2 poles (-20.4394, -11.4919) (-20.6823, -11.2696) (-21.4397, -10.9402) (-21.8555, -10.9402) knots 0 0 0 1 2 2 2
  spline S135 degree 2 poles (-21.8555, -10.9402) (-22.3248, -10.9402) (-22.9053, -11.3807) (-22.9053, -11.7389) knots 0 0 0 1 2 2 2
  spline S136 degree 2 poles (-22.9053, -11.7389) (-22.9053, -12.06) (-22.5636, -12.4428) (-22.2425, -12.5293) knots 0 0 0 1 2 2 2
  spline S137 degree 2 poles (-22.2425, -12.5293) (-22.0284, -12.5869) (-21.4068, -12.7351) (-21.201, -12.7969) knots 0 0 0 1 2 2 2
  spline S138 degree 2 poles (-21.201, -12.7969) (-20.6782, -12.9574) (-20.1924, -13.6037) (-20.1924, -14.0771) knots 0 0 0 1 2 2 2
  spline S139 degree 2 poles (-20.1924, -14.0771) (-20.1924, -14.3777) (-20.4353, -14.954) (-20.6535, -15.1557) knots 0 0 0 1 2 2 2
  spline S140 degree 2 poles (-20.6535, -15.1557) (-20.8963, -15.378) (-21.5138, -15.6168) (-21.979, -15.6168) knots 0 0 0 1 2 2 2
  line L143 (-16.5615, -15.5262) -> (-17.2037, -15.5262)
  line L144 (-17.2037, -15.5262) -> (-17.2037, -13.3526)
  spline S141 degree 2 poles (-17.2037, -13.3526) (-17.2037, -13.0891) (-17.2531, -12.6363) (-17.3272, -12.5005) knots 0 0 0 1 2 2 2
  spline S142 degree 2 poles (-17.3272, -12.5005) (-17.4054, -12.3564) (-17.6853, -12.2164) (-17.9241, -12.2164) knots 0 0 0 1 2 2 2
  spline S143 degree 2 poles (-17.9241, -12.2164) (-18.1629, -12.2164) (-18.6692, -12.4716) (-18.9121, -12.6775) knots 0 0 0 1 2 2 2
  line L145 (-18.9121, -12.6775) -> (-18.9121, -15.5262)
  line L146 (-18.9121, -15.5262) -> (-19.5543, -15.5262)
  line L147 (-19.5543, -15.5262) -> (-19.5543, -10.2198)
  line L148 (-19.5543, -10.2198) -> (-18.9121, -10.2198)
  line L149 (-18.9121, -10.2198) -> (-18.9121, -12.1382)
  spline S144 degree 2 poles (-18.9121, -12.1382) (-18.6239, -11.8788) (-18.0682, -11.6071) (-17.7553, -11.6071) knots 0 0 0 1 2 2 2
  spline S145 degree 2 poles (-17.7553, -11.6071) (-17.1954, -11.6071) (-16.5615, -12.3481) (-16.5615, -13.0521) knots 0 0 0 1 2 2 2
  line L150 (-16.5615, -13.0521) -> (-16.5615, -15.5262)
  spline S146 degree 2 poles (-13.5357, -15.1228) (-13.6139, -15.1804) (-13.8774, -15.3863) (-14.0009, -15.448) knots 0 0 0 1 2 2 2
  spline S147 degree 2 poles (-14.0009, -15.448) (-14.1697, -15.5386) (-14.4866, -15.6333) (-14.7748, -15.6333) knots 0 0 0 1 2 2 2
  spline S148 degree 2 poles (-14.7748, -15.6333) (-15.0095, -15.6333) (-15.4335, -15.4562) (-15.594, -15.2957) knots 0 0 0 1 2 2 2
  spline S149 degree 2 poles (-15.594, -15.2957) (-15.7464, -15.1393) (-15.9316, -14.6782) (-15.9316, -14.4229) knots 0 0 0 1 2 2 2
  spline S150 degree 2 poles (-15.9316, -14.4229) (-15.9316, -14.0277) (-15.5982, -13.4679) (-15.2359, -13.3073) knots 0 0 0 1 2 2 2
  spline S151 degree 2 poles (-15.2359, -13.3073) (-14.9148, -13.1591) (-14.042, -13.048) (-13.5357, -13.0192) knots 0 0 0 1 2 2 2
  line L151 (-13.5357, -13.0192) -> (-13.5357, -12.8957)
  spline S152 degree 2 poles (-13.5357, -12.8957) (-13.5357, -12.6734) (-13.6715, -12.3975) (-13.795, -12.3193) knots 0 0 0 1 2 2 2
  spline S153 degree 2 poles (-13.795, -12.3193) (-13.9185, -12.2411) (-14.2726, -12.1917) (-14.4619, -12.1917) knots 0 0 0 1 2 2 2
  spline S154 degree 2 poles (-14.4619, -12.1917) (-14.6842, -12.1917) (-15.2853, -12.3234) (-15.5858, -12.4511) knots 0 0 0 1 2 2 2
  line L152 (-15.5858, -12.4511) -> (-15.6229, -12.4511)
  line L153 (-15.6229, -12.4511) -> (-15.6229, -11.7965)
  spline S155 degree 2 poles (-15.6229, -11.7965) (-15.4458, -11.7471) (-14.783, -11.6236) (-14.4578, -11.6236) knots 0 0 0 1 2 2 2
  spline S156 degree 2 poles (-14.4578, -11.6236) (-14.0626, -11.6236) (-13.5233, -11.7471) (-13.3093, -11.9076) knots 0 0 0 1 2 2 2
  spline S157 degree 2 poles (-13.3093, -11.9076) (-13.0993, -12.0641) (-12.8935, -12.5622) (-12.8935, -12.9204) knots 0 0 0 1 2 2 2
  line L154 (-12.8935, -12.9204) -> (-12.8935, -15.5262)
  line L155 (-12.8935, -15.5262) -> (-13.5357, -15.5262)
  line L156 (-13.5357, -15.5262) -> (-13.5357, -15.1228)
  line L157 (-13.5357, -14.5876) -> (-13.5357, -13.5296)
  spline S158 degree 2 poles (-13.5357, -13.5296) (-13.7662, -13.5502) (-14.4619, -13.6202) (-14.6801, -13.6861) knots 0 0 0 1 2 2 2
  spline S159 degree 2 poles (-14.6801, -13.6861) (-14.9354, -13.7643) (-15.2688, -14.0895) (-15.2688, -14.3777) knots 0 0 0 1 2 2 2
  spline S160 degree 2 poles (-15.2688, -14.3777) (-15.2688, -14.707) (-14.8983, -15.0405) (-14.5443, -15.0405) knots 0 0 0 1 2 2 2
  spline S161 degree 2 poles (-14.5443, -15.0405) (-14.2438, -15.0405) (-13.7498, -14.7811) (-13.5357, -14.5876) knots 0 0 0 1 2 2 2
  line L158 (-9.9871, -10.8373) -> (-10.02, -10.8373)
  spline S162 degree 2 poles (-10.02, -10.8373) (-10.1065, -10.8044) (-10.4276, -10.7467) (-10.5552, -10.7467) knots 0 0 0 1 2 2 2
  spline S163 degree 2 poles (-10.5552, -10.7467) (-10.9586, -10.7467) (-11.3044, -11.109) (-11.3044, -11.5865) knots 0 0 0 1 2 2 2
  line L159 (-11.3044, -11.5865) -> (-11.3044, -11.7142)
  line L160 (-11.3044, -11.7142) -> (-10.2423, -11.7142)
  line L161 (-10.2423, -11.7142) -> (-10.2423, -12.2452)
  line L162 (-10.2423, -12.2452) -> (-11.2839, -12.2452)
  line L163 (-11.2839, -12.2452) -> (-11.2839, -15.5262)
  line L164 (-11.2839, -15.5262) -> (-11.9261, -15.5262)
  line L165 (-11.9261, -15.5262) -> (-11.9261, -12.2452)
  line L166 (-11.9261, -12.2452) -> (-12.3583, -12.2452)
  line L167 (-12.3583, -12.2452) -> (-12.3583, -11.7142)
  line L168 (-12.3583, -11.7142) -> (-11.9261, -11.7142)
  line L169 (-11.9261, -11.7142) -> (-11.9261, -11.5865)
  spline S164 degree 2 poles (-11.9261, -11.5865) (-11.9261, -10.9032) (-11.2633, -10.1869) (-10.6458, -10.1869) knots 0 0 0 1 2 2 2
  spline S165 degree 2 poles (-10.6458, -10.1869) (-10.4688, -10.1869) (-10.1271, -10.2239) (-9.9871, -10.2486) knots 0 0 0 1 2 2 2
  line L170 (-9.9871, -10.2486) -> (-9.9871, -10.8373)
  spline S166 degree 2 poles (-8.468, -15.6003) (-8.9909, -15.6003) (-9.5795, -15.0034) (-9.5795, -14.3571) knots 0 0 0 1 2 2 2
  line L171 (-9.5795, -14.3571) -> (-9.5795, -12.2452)
  line L172 (-9.5795, -12.2452) -> (-10.0118, -12.2452)
  line L173 (-10.0118, -12.2452) -> (-10.0118, -11.7142)
  line L174 (-10.0118, -11.7142) -> (-9.5795, -11.7142)
  line L175 (-9.5795, -11.7142) -> (-9.5795, -10.6191)
  line L176 (-9.5795, -10.6191) -> (-8.9373, -10.6191)
  line L177 (-8.9373, -10.6191) -> (-8.9373, -11.7142)
  line L178 (-8.9373, -11.7142) -> (-7.7559, -11.7142)
  line L179 (-7.7559, -11.7142) -> (-7.7559, -12.2452)
  line L180 (-7.7559, -12.2452) -> (-8.9373, -12.2452)
  line L181 (-8.9373, -12.2452) -> (-8.9373, -14.0607)
  spline S167 degree 2 poles (-8.9373, -14.0607) (-8.9373, -14.3488) (-8.9168, -14.6658) (-8.8468, -14.8017) knots 0 0 0 1 2 2 2
  spline S168 degree 2 poles (-8.8468, -14.8017) (-8.7891, -14.9211) (-8.5298, -15.0405) (-8.3075, -15.0405) knots 0 0 0 1 2 2 2
  spline S169 degree 2 poles (-8.3075, -15.0405) (-8.1511, -15.0405) (-7.8588, -14.9458) (-7.7929, -14.917) knots 0 0 0 1 2 2 2
  line L182 (-7.7929, -14.917) -> (-7.7559, -14.917)
  line L183 (-7.7559, -14.917) -> (-7.7559, -15.4933)
  spline S170 degree 2 poles (-7.7559, -15.4933) (-7.937, -15.5427) (-8.3075, -15.6003) (-8.468, -15.6003) knots 0 0 0 1 2 2 2
  line L184 (-1.3667, -10.4462) -> (-3.1163, -15.5262)
  line L185 (-3.1163, -15.5262) -> (-3.845, -15.5262)
  line L186 (-3.845, -15.5262) -> (-5.5946, -10.4462)
  line L187 (-5.5946, -10.4462) -> (-4.87, -10.4462)
  line L188 (-4.87, -10.4462) -> (-3.4621, -14.6658)
  line L189 (-3.4621, -14.6658) -> (-2.0542, -10.4462)
  line L190 (-2.0542, -10.4462) -> (-1.3667, -10.4462)
  spline S171 degree 2 poles (2.1942, -12.9862) (2.1942, -14.353) (1.3997, -15.6333) (0.5722, -15.6333) knots 0 0 0 1 2 2 2
  spline S172 degree 2 poles (0.5722, -15.6333) (-0.2676, -15.6333) (-1.0539, -14.3283) (-1.0539, -12.9903) knots 0 0 0 1 2 2 2
  spline S173 degree 2 poles (-1.0539, -12.9903) (-1.0539, -11.6154) (-0.2594, -10.3433) (0.5722, -10.3433) knots 0 0 0 1 2 2 2
  spline S174 degree 2 poles (0.5722, -10.3433) (1.4079, -10.3433) (2.1942, -11.6606) (2.1942, -12.9862) knots 0 0 0 1 2 2 2
  spline S175 degree 2 poles (1.3215, -14.5341) (1.4203, -14.283) (1.5026, -13.509) (1.5026, -12.9862) knots 0 0 0 1 2 2 2
  spline S176 degree 2 poles (1.5026, -12.9862) (1.5026, -12.4634) (1.4203, -11.6936) (1.3173, -11.4342) knots 0 0 0 1 2 2 2
  spline S177 degree 2 poles (1.3173, -11.4342) (1.2144, -11.1749) (0.8563, -10.9073) (0.5722, -10.9073) knots 0 0 0 1 2 2 2
  spline S178 degree 2 poles (0.5722, -10.9073) (0.2882, -10.9073) (-0.0782, -11.1749) (-0.1853, -11.4425) knots 0 0 0 1 2 2 2
  spline S179 degree 2 poles (-0.1853, -11.4425) (-0.2882, -11.7018) (-0.3623, -12.4922) (-0.3623, -12.9903) knots 0 0 0 1 2 2 2
  spline S180 degree 2 poles (-0.3623, -12.9903) (-0.3623, -13.5255) (-0.2964, -14.2418) (-0.1894, -14.5217) knots 0 0 0 1 2 2 2
  spline S181 degree 2 poles (-0.1894, -14.5217) (-0.0906, -14.7852) (0.2758, -15.0693) (0.5722, -15.0693) knots 0 0 0 1 2 2 2
  spline S182 degree 2 poles (0.5722, -15.0693) (0.8522, -15.0693) (1.2185, -14.8017) (1.3215, -14.5341) knots 0 0 0 1 2 2 2
  line L191 (5.7222, -15.5262) -> (3.244, -15.5262)
  line L192 (3.244, -15.5262) -> (3.244, -15.0075)
  line L193 (3.244, -15.0075) -> (4.1661, -15.0075)
  line L194 (4.1661, -15.0075) -> (4.1661, -11.603)
  line L195 (4.1661, -11.603) -> (3.244, -11.603)
  line L196 (3.244, -11.603) -> (3.244, -11.1378)
  spline S183 degree 2 poles (3.244, -11.1378) (3.7668, -11.1378) (4.2608, -10.8414) (4.2937, -10.4298) knots 0 0 0 1 2 2 2
  line L197 (4.2937, -10.4298) -> (4.8206, -10.4298)
  line L198 (4.8206, -10.4298) -> (4.8206, -15.0075)
  line L199 (4.8206, -15.0075) -> (5.7222, -15.0075)
  line L200 (5.7222, -15.0075) -> (5.7222, -15.5262)
  spline S184 degree 2 poles (12.1936, -11.9776) (12.1936, -12.307) (11.959, -12.8998) (11.749, -13.1056) knots 0 0 0 1 2 2 2
  spline S185 degree 2 poles (11.749, -13.1056) (11.4856, -13.365) (10.7734, -13.6325) (10.23, -13.6325) knots 0 0 0 1 2 2 2
  line L201 (10.23, -13.6325) -> (9.6578, -13.6325)
  line L202 (9.6578, -13.6325) -> (9.6578, -15.5262)
  line L203 (9.6578, -15.5262) -> (8.9826, -15.5262)
  line L204 (8.9826, -15.5262) -> (8.9826, -10.4462)
  line L205 (8.9826, -10.4462) -> (10.2588, -10.4462)
  spline S186 degree 2 poles (10.2588, -10.4462) (10.7116, -10.4462) (11.3456, -10.5944) (11.5885, -10.7632) knots 0 0 0 1 2 2 2
  spline S187 degree 2 poles (11.5885, -10.7632) (11.8725, -10.9567) (12.1936, -11.5536) (12.1936, -11.9776) knots 0 0 0 1 2 2 2
  spline S188 degree 2 poles (11.4897, -11.9982) (11.4897, -11.7347) (11.3086, -11.3478) (11.1233, -11.2243) knots 0 0 0 1 2 2 2
  spline S189 degree 2 poles (11.1233, -11.2243) (10.9628, -11.1172) (10.5346, -11.0308) (10.2176, -11.0308) knots 0 0 0 1 2 2 2
  line L206 (10.2176, -11.0308) -> (9.6578, -11.0308)
  line L207 (9.6578, -11.0308) -> (9.6578, -13.0562)
  line L208 (9.6578, -13.0562) -> (10.1188, -13.0562)
  spline S190 degree 2 poles (10.1188, -13.0562) (10.5305, -13.0562) (11.0369, -12.9245) (11.2015, -12.7516) knots 0 0 0 1 2 2 2
  spline S191 degree 2 poles (11.2015, -12.7516) (11.3538, -12.5993) (11.4897, -12.2411) (11.4897, -11.9982) knots 0 0 0 1 2 2 2
  line L209 (16.5203, -10.4462) -> (14.7707, -15.5262)
  line L210 (14.7707, -15.5262) -> (14.042, -15.5262)
  line L211 (14.042, -15.5262) -> (12.2924, -10.4462)
  line L212 (12.2924, -10.4462) -> (13.017, -10.4462)
  line L213 (13.017, -10.4462) -> (14.4249, -14.6658)
  line L214 (14.4249, -14.6658) -> (15.8328, -10.4462)
  line L215 (15.8328, -10.4462) -> (16.5203, -10.4462)
  spline S192 degree 2 poles (20.0812, -12.9862) (20.0812, -14.353) (19.2867, -15.6333) (18.4593, -15.6333) knots 0 0 0 1 2 2 2
  spline S193 degree 2 poles (18.4593, -15.6333) (17.6194, -15.6333) (16.8332, -14.3283) (16.8332, -12.9903) knots 0 0 0 1 2 2 2
  spline S194 degree 2 poles (16.8332, -12.9903) (16.8332, -11.6154) (17.6277, -10.3433) (18.4593, -10.3433) knots 0 0 0 1 2 2 2
  spline S195 degree 2 poles (18.4593, -10.3433) (19.2949, -10.3433) (20.0812, -11.6606) (20.0812, -12.9862) knots 0 0 0 1 2 2 2
  spline S196 degree 2 poles (19.2085, -14.5341) (19.3073, -14.283) (19.3896, -13.509) (19.3896, -12.9862) knots 0 0 0 1 2 2 2
  spline S197 degree 2 poles (19.3896, -12.9862) (19.3896, -12.4634) (19.3073, -11.6936) (19.2044, -11.4342) knots 0 0 0 1 2 2 2
  spline S198 degree 2 poles (19.2044, -11.4342) (19.1015, -11.1749) (18.7433, -10.9073) (18.4593, -10.9073) knots 0 0 0 1 2 2 2
  spline S199 degree 2 poles (18.4593, -10.9073) (18.1752, -10.9073) (17.8088, -11.1749) (17.7018, -11.4425) knots 0 0 0 1 2 2 2
  spline S200 degree 2 poles (17.7018, -11.4425) (17.5989, -11.7018) (17.5248, -12.4922) (17.5248, -12.9903) knots 0 0 0 1 2 2 2
  spline S201 degree 2 poles (17.5248, -12.9903) (17.5248, -13.5255) (17.5906, -14.2418) (17.6977, -14.5217) knots 0 0 0 1 2 2 2
  spline S202 degree 2 poles (17.6977, -14.5217) (17.7965, -14.7852) (18.1629, -15.0693) (18.4593, -15.0693) knots 0 0 0 1 2 2 2
  spline S203 degree 2 poles (18.4593, -15.0693) (18.7392, -15.0693) (19.1056, -14.8017) (19.2085, -14.5341) knots 0 0 0 1 2 2 2
  line L216 (23.6092, -15.5262) -> (21.131, -15.5262)
  line L217 (21.131, -15.5262) -> (21.131, -15.0075)
  line L218 (21.131, -15.0075) -> (22.0531, -15.0075)
  line L219 (22.0531, -15.0075) -> (22.0531, -11.603)
  line L220 (22.0531, -11.603) -> (21.131, -11.603)
  line L221 (21.131, -11.603) -> (21.131, -11.1378)
  spline S204 degree 2 poles (21.131, -11.1378) (21.6538, -11.1378) (22.1478, -10.8414) (22.1807, -10.4298) knots 0 0 0 1 2 2 2
  line L222 (22.1807, -10.4298) -> (22.7077, -10.4298)
  line L223 (22.7077, -10.4298) -> (22.7077, -15.0075)
  line L224 (22.7077, -15.0075) -> (23.6092, -15.0075)
  line L225 (23.6092, -15.0075) -> (23.6092, -15.5262)
  point P0 (0, 19.05)
  constraints: 2 end point, 2 midpoint, 1 horizontal
emboss "Emboss1" sketch "Sketch4" operation cut depth 2.54 direction (-1, 0, 0) wrap yes faces at (-12.6588, 1.0219, -25.4)
equation "\"d0\" = hexSize"
equation "\"d1\" = length"
equation "\"d6\" = printOffset"
equation "\"hexSize\" = 19.05"
equation "\"length\" = 38.1"
equation "\"printOffset\" = 0.1905"
body "Solid1"
